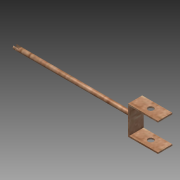
# Autodesk Inventor part: 顶杆
Saved by Autodesk Inventor 2013 (Build 170138000, 138)
## iProperties
Created: 2012-09-25
Part Number: 顶杆
Material: 木材(桦木)
Document SubType Name: Modeling
Designer: Zhensheng
Density: 1 g/cm^3
Mass: 0.249746 g
Surface Area: 5.11372 cm^2
Volume: 0.249746 cm^3
Author: Zhensheng
Autodesk Inventor part; units mm, degrees
ref_plane "YZ Plane" through (0, 0, 0) normal (1, 0, 0) x (0, 1, 0)
ref_plane "XZ Plane" through (0, 0, 0) normal (0, 1, 0) x (-1, 0, 0)
ref_plane "XY Plane" through (0, 0, 0) normal (0, 0, 1) x (1, 0, 0)
sketch "草图1" plane through (0, 0, 0) normal (1, 0, 0) x (0, 1, 0)
  circle A0 centre (0, 0) radius 1.5
  dimension "杆直径" = 3
  constraints: 1 centre point, 1 coincident
  measures "杆直径" diameter of A0
extrude "拉伸1" add sketch "草图1" along normal blind 84
sketch "草图2" plane through (84, 0, 0) normal (1, 0, 0) x (0, 0, -1)
  line L0 (10, -5) -> (-10, -5)
  line L1 (-10, -5) -> (-10, 5)
  line L2 (-10, 5) -> (10, 5)
  line L3 (10, 5) -> (10, -5)
  line L4 (10, -5) -> (-10, 5) construction
  line L5 (-10, -5) -> (10, 5) construction
  point P0 (0, 0)
  dimension "框长" = 20
  dimension "框宽" = 10
  constraints: 12 end point, 2 horizontal, 2 midpoint, 2 vertical
  measures "框长" distance of L1.end L2.end
  measures "框宽" distance of L0.end L1.end
extrude "拉伸2" add sketch "草图2" along normal blind 1
sketch "草图3" plane through (85, 0, 0) normal (1, 0, 0) x (0, 0, -1)
  line L0 (-10, -5) -> (10, -5) projected
  line L1 (10, -5) -> (10, 5) projected
  line L2 (10, 5) -> (-10, 5) projected
  line L3 (-10, 5) -> (-10, -5) projected
  line L4 (-10, 5) -> (-9, 5)
  line L5 (-9, 5) -> (-9, -5)
  line L6 (10, 5) -> (9, 5)
  line L7 (9, 5) -> (9, -5)
  point P0 (0, 0)
  dimension "d7" = 1
  dimension "d8" = 1
  constraints: 8 end point, 4 point on line
  measures "d7" distance of L2.end L4.end
  measures "d8" distance of L1.end L6.end
extrude "拉伸3" add sketch "草图3" along normal blind 20 contours L3 L2 L5 L0 | L7 L2 L1 L0
hole "孔1" at (95, 0, -10) direction (0, 0, 1) diameter 4 end through all
sketch "草图5" plane through (0, 0, 0) normal (0, 0, 1) x (1, 0, 0)
  line L0 (0, 1.5) -> (0, -1.5) projected
  line L1 (0, 1.5) -> (84, 1.5) projected
  line L2 (0, -1.5) -> (84, -1.5) projected
  line L3 (0, 1) -> (4, 1)
  line L4 (4, 1) -> (4, -1)
  line L5 (4, -1) -> (0, -1)
  line L6 (0, 0) -> (4, 0) construction
  point P0 (2, 0)
  dimension "d21" = 4
  dimension "宽度" = 2
  constraints: 8 end point, 2 midpoint, 2 point on line, 1 horizontal, 1 other
  measures "d21" distance of L3.start L3.end
  measures "宽度" distance between parallel lines of L5 L3
extrude "拉伸4" cut sketch "草图5" along normal through all both and the other way through all
sketch "草图6" plane through (0, 0, 0) normal (0, 1, 0) x (-1, 0, 0)
  line L0 (-4, 1.5) -> (-84, 1.5) projected
  line L1 (-4, -1.5) -> (-84, -1.5) projected
  line L2 (0, 1.118) -> (0, -1.118) projected
  line L3 (-4, -1.118) -> (-4, 1.118) projected
  circle A0 centre (-2, 0) radius 0.5
  point P0 (0, 0)
  dimension "位置1" = 2
  dimension "位置2" = 1.5
  dimension "销孔径" = 1
  constraints: 1 centre point, 1 coincident
  measures "位置1" distance from line of point (-2, 0) L2
  measures "位置2" distance from line of point (-2, 0) L0
  measures "销孔径" diameter of A0
extrude "拉伸5" cut sketch "草图6" along normal mid plane 10
